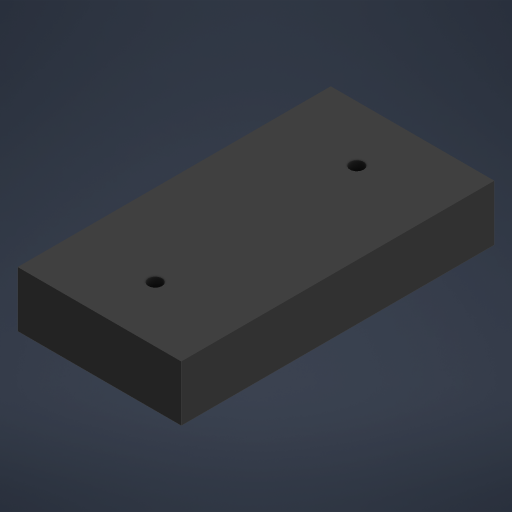
# Autodesk Inventor part: battery_case
Saved by Autodesk Inventor 2023 (Build 270158000, 158)
## iProperties
Created: 2022-12-04
Part Number: battery_case
Material: Generic
Document SubType Name: Modeling
Designer: jeff7
Density: 1 g/cm^3
Appearance: Default
Author: jeff7
Autodesk Inventor part; units mm, degrees
ref_plane "YZ Plane" through (0, 0, 0) normal (1, 0, 0) x (0, 1, 0)
ref_plane "XZ Plane" through (0, 0, 0) normal (0, 1, 0) x (-1, 0, 0)
ref_plane "XY Plane" through (0, 0, 0) normal (0, 0, 1) x (1, 0, 0)
sketch "bat_base" plane through (0, 0, 0) normal (0, 1, 0) x (-1, 0, 0)
  line L0 (23.5, 45) -> (-23.5, 45)
  line L1 (-23.5, 45) -> (-23.5, -45)
  line L2 (-23.5, -45) -> (23.5, -45)
  line L3 (23.5, -45) -> (23.5, 45)
  circle A0 centre (0, 29) radius 2
  circle A1 centre (0, -29) radius 2
  point P0 (0, 0)
  point P1 (-23.5, 0)
  point P2 (0, -45)
  point P3 (0, 45)
  dimension "d0" = 47
  dimension "d1" = 90
  dimension "d2" = 4
  dimension "d3" = 16
  dimension "d4" = 4
  dimension "d5" = 16
  constraints: 8 end point, 3 midpoint, 3 vertical alignment, 2 centre point, 2 parallel, 1 horizontal, 1 horizontal alignment, 1 perpendicular
  measures "d0" distance of L2.end L1.end
  measures "d1" distance of L1.end L0.end
  measures "d2" diameter of A0
  measures "d3" distance from line of L0 A0.centre
  measures "d4" diameter of A1
  measures "d5" distance from line of L2 A1.centre
extrude "bat_block" add sketch "bat_base" along normal blind 16
body "Solid1"
